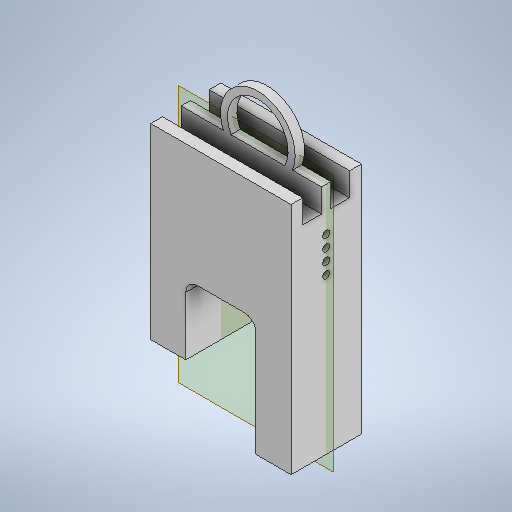
# Autodesk Inventor part: support balise
Saved by Autodesk Inventor 2025.2 (Build 292293000, 293)
## iProperties
Created: 2025-03-18
Part Number: support balise
Material: Generic
Document SubType Name: Modeling
Designer: elear
Density: 1 g/cm^3
Appearance: Default
Author: elear
## iProperties of the stored document support balise_3DPrint.ipt
Created: 2025-03-18
Part Number: support balise_3DPrint
Material: Generic
Document SubType Name: Modeling
Designer: elear
Density: 1 g/cm^3
Appearance: Default
Author: elear
Autodesk Inventor part; units mm, degrees
ref_plane "YZ Plane" through (0, 0, 0) normal (1, 0, 0) x (0, 1, 0)
ref_plane "XZ Plane" through (0, 0, 0) normal (0, 1, 0) x (-1, 0, 0)
ref_plane "XY Plane" through (0, 0, 0) normal (0, 0, 1) x (1, 0, 0)
sketch "Sketch1" plane through (0, 0, 0) normal (0, 1, 0) x (-1, 0, 0)
  line L0 (18.599, 14.3602) -> (-41.401, 14.3602)
  line L1 (-41.401, 14.3602) -> (-41.401, -15.6398)
  line L2 (-41.401, -15.6398) -> (18.599, -15.6398)
  line L3 (18.599, -15.6398) -> (18.599, 14.3602)
  line L4 (18.599, 9.3602) -> (-41.401, 9.3602)
  line L5 (18.599, 1.3602) -> (-41.401, 1.3602)
  line L6 (18.599, -2.6398) -> (-41.401, -2.6398)
  line L7 (18.599, -10.6398) -> (-41.401, -10.6398)
  line L8 (-11.401, 14.3602) -> (-11.401, 9.3602)
  line L9 (-11.401, -10.6398) -> (-11.401, -15.6398)
  circle A0 centre (-11.401, 5.3602) radius 1.5
  circle A1 centre (-11.401, -6.6398) radius 1.5
  line L10 (-11.401, 9.3602) -> (-11.401, 1.3602)
  line L11 (-11.401, -2.6398) -> (-11.401, 1.3602)
  line L12 (-11.401, -2.6398) -> (-11.401, -10.6398)
  line L13 (-11.401, 5.3602) -> (-11.401, 9.3602)
  line L14 (-11.401, -6.6398) -> (-11.401, -10.6398)
  line L15 (3.599, 14.3602) -> (3.599, -15.6398)
  line L16 (-26.401, 14.3602) -> (-26.401, -15.6398)
  point P0 (0, 0)
  point P1 (-11.401, -13.1398)
  dimension "d0" = 30
  dimension "d1" = 60
  dimension "d2" = 8
  dimension "d3" = 4
  dimension "d4" = 4
  dimension "d5" = 3
  dimension "d6" = 30
  dimension "d13" = 30
  dimension "d14" = 15
  dimension "d15" = 15
  dimension "d20" = 5
  constraints: 34 end point, 12 point on line, 8 midpoint, 7 collinear, 7 perpendicular, 2 centre point, 2 parallel, 1 equal radius, 1 horizontal
  measures "d0" distance of L2.end L0.start
  measures "d1" distance of L0.start L0.end
  measures "d2" distance between parallel lines of L5 L4
  measures "d3" distance of L8.end point (-11.401, 5.36)
  measures "d4" distance of L8.end L13.start
  measures "d5" diameter of A0
  measures "d6" distance between parallel lines of L1 L8
  measures "d13" distance between parallel lines of L16 L15
  measures "d14" distance between parallel lines of L1 L16
  measures "d15" distance from line of L16 point (-11.401, -13.14)
  measures "d20" distance between parallel lines of L4 L0
extrude "Extrusion1" add sketch "Sketch1" against normal blind 30 contours L3 L4 L15 L0 | L3 L5 L15 L4 | L3 L6 L15 L5 | L3 L7 L15 L6 | L3 L2 L15 L7
extrude "Extrusion2" add sketch "Sketch1" against normal blind 50 contours L16 L4 L1 L0 | L16 L5 L1 L4 | L16 L6 L1 L5 | L16 L7 L1 L6 | L16 L2 L1 L7
extrude "Extrusion3" add sketch "Sketch1" along normal blind 40
extrude "Extrusion4" cut sketch "Sketch1" along normal blind 40 contours L10 A0 | A0 L10 | L12 A1 | A1 L12
extrude "Extrusion5" add sketch "Sketch1" along normal blind 10 from surface at 40 contours L3 L4 L15 L0 | L15 L4 L8 L0 | L8 L4 L16 L0 | L3 L6 L15 L5 | L16 L4 L1 L0 | L15 L6 L11 L5 | L11 L6 L16 L5 | L3 L2 L15 L7 | L16 L6 L1 L5 | L15 L2 L9 L7 | L9 L2 L16 L7 | L16 L2 L1 L7
sketch "Sketch3" plane through (0, 40, 0) normal (0, 1, 0) x (1, 0, 0)
  circle A0 centre (-8.599, -6.3602) radius 1.5
  circle A1 centre (-8.599, 6.6398) radius 1.5037
  circle A2 centre (31.401, -6.3602) radius 1.372
  circle A3 centre (31.401, 6.6398) radius 1.4081
  line L0 (-8.599, -6.3602) -> (-8.599, 6.6398)
  line L1 (-8.599, 6.6398) -> (31.401, 6.6398)
  line L2 (31.401, 6.6398) -> (31.401, -6.3602)
  line L3 (31.401, -6.3602) -> (-8.599, -6.3602)
  line L4 (-18.599, -1.3602) -> (-18.599, -9.3602) projected
  line L5 (41.401, 2.6398) -> (41.401, 10.6398) projected
  line L6 (41.401, -14.3602) -> (-18.599, -14.3602) projected
  point P0 (0, 0)
  dimension "d21" = 3
  dimension "d23" = 10
  dimension "d24" = 13
  dimension "d25" = 10
  dimension "d26" = 8
  constraints: 8 end point, 4 centre point, 2 perpendicular, 1 parallel, 1 vertical
  measures "d21" diameter of A0
  measures "d23" distance from line of L4 L0.start
  measures "d24" distance of L1.end L2.end
  measures "d25" distance between parallel lines of L5 L2
  measures "d26" distance between parallel lines of L6 L3
hole "Hole1" at (-8.599, 40, -6.6398) at (-8.599, 40, 6.3602) at (31.401, 40, 6.3602) at (31.401, 40, -6.6398) direction (0, -1, 0) diameter 3 end through all countersink diameter 3.5 countersink angle 80
sketch "Sketch4" plane through (0, 0, 0) normal (0, -1, 0) x (1, 0, 0)
  circle A0 centre (11.401, 5.3602) radius 1.5 projected
  circle A1 centre (11.401, -6.6398) radius 1.5 projected
  line L0 (-3.599, 14.3602) -> (-3.599, -15.6398) projected
  line L1 (26.401, -15.6398) -> (-3.599, -15.6398) projected
  line L2 (26.401, -15.6398) -> (26.401, 14.3602) projected
  line L3 (-3.599, 14.3602) -> (26.401, 14.3602) projected
  circle A2 centre (11.401, 5.3602) radius 6
  circle A3 centre (11.401, -6.6398) radius 6
  point P0 (0, 0)
  point P1 (11.401, -0.6398)
  dimension "d34" = 12
  dimension "d35" = 12
  constraints: 2 centre point, 2 coincident
  measures "d34" diameter of A2
  measures "d35" diameter of A3
extrude "Extrusion6" cut sketch "Sketch4" against normal blind 30 contours A2 | A3
loft "Loft1" cut section 1 edges at (12.901, 40, -6.6398) section 2 edges at (15.6436, 30, -2.3971) (7.1584, 30, -10.8824)
loft "Loft2" cut section 1 edges at (12.901, 40, 5.3602) section 2 edges at (15.6436, 30, 1.1176) (7.1584, 30, 9.6029)
fillet "Fillet1" radius 5 2 edges at (-3.599, 0, -0.6398) (26.401, 0, -0.6398)
sketch "Sketch5" plane through (41.401, -50, 14.3602) normal (1, 0, 0) x (0, 0, -1)
  circle A0 centre (15, 81.5) radius 1.5
  line L0 (27, 80) -> (15, 80) projected
  line L1 (15, 50) -> (15, 80) projected
  circle A1 centre (15, 76.5) radius 1.5
  circle A2 centre (15, 71.5) radius 1.5
  circle A3 centre (15, 66.5) radius 1.5
  point P0 (14.3602, 50)
  dimension "d47" = 3
  dimension "d48" = 3
  dimension "d49" = 3
  dimension "d50" = 3
  dimension "d51" = 5
  dimension "d52" = 5
  dimension "d53" = 5
  constraints: 3 centre point, 1 horizontal, 1 point on line, 1 vertical alignment, 1 other
  measures "d48" diameter of A1
  measures "d49" diameter of A2
  measures "d50" diameter of A3
  measures "d51" distance of A1.centre point (15, 81.5)
  measures "d52" distance of A2.centre A1.centre
  measures "d53" distance of A3.centre A2.centre
extrude "Extrusion7" cut sketch "Sketch5" against normal blind 5
sketch "Sketch6" plane through (41.401, 50, -2.6398) normal (0, 0, -1) x (-1, 0, 0)
  point P0 (41.401, -50)
sketch "Sketch7" plane through (-3.599, -30, -15.6398) normal (0, 0, -1) x (-1, 0, 0)
  line L0 (-21, 30) -> (-21, 60) projected
  line L1 (0, 25) -> (0, 0) projected
  line L2 (15, 0) -> (0, 0) projected
  line L3 (15, 0) -> (15, 80) projected
  line L4 (15, 80) -> (-45, 80) projected
  line L5 (-45, -20) -> (-45, 80) projected
  line L6 (-30, -20) -> (-45, -20) projected
  line L7 (-30, 25) -> (-30, -20) projected
  arc A0 (-25, 30) -> (-30, 25) centre (-25, 25) ccw projected
  line L8 (-25, 30) -> (-5, 30) projected
  arc A1 (0, 25) -> (-5, 30) centre (-5, 25) ccw projected
  line L9 (-45, 80) -> (15, 80) projected
  circle A2 centre (-17.7825, 85.9524) radius 15.9524
  line L10 (-45, 70) -> (15, 70) projected
  circle A3 centre (-17.7825, 85.9524) radius 12.9546
  point P0 (-3.599, 30)
  point P1 (-29.2886, 80)
  point P2 (-6.2763, 80)
  point P3 (-2.9822, 80)
  point P4 (-32.5827, 80)
  constraints: 2 centre point, 1 coincident, 1 tangent
ref_plane "Work Plane1" through (-3.599, -30, -0.6398) normal (0, 0, -1) x (-1, 0, 0)
extrude "Extrusion9" add sketch "Sketch7" along normal mid plane 4 from surface at -15 contours L4 A3 A2 picked at (-2.9754, 87.1902)
body "Solid1"
